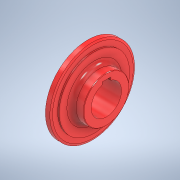
# Autodesk Inventor part: звездочка
Saved by Autodesk Inventor 2021 (Build 250183000, 183)
## iProperties
Created: 2023-04-24
Part Number: звездочка
Material: Сталь, углеродистая
Document SubType Name: Modeling
Designer: gdevc
Density: 7.85 g/cm^3
Appearance: Светло-красный
Mass: 4605.53 g
Surface Area: 813.785 cm^2
Volume: 586.691 cm^3
Author: gdevc
Autodesk Inventor part; units mm, degrees
ref_plane "YZ Plane" through (0, 0, 0) normal (1, 0, 0) x (0, 1, 0)
ref_plane "XY Plane" through (0, 0, 0) normal (0, 0, 1) x (1, 0, 0)
sketch "Эскиз1" plane through (0, 0, 0) normal (0, 0, 1) x (1, 0, 0)
  line L0 (0, 32.5) -> (70, 32.5)
  line L1 (0, 0) -> (109.6934, 0)
  line L2 (0, 32.5) -> (0, 44.804)
  line L3 (35, 68.0113) -> (35, 17.7812) construction
  line L4 (0, 80) -> (70, 80) construction
  line L5 (70, 32.5) -> (0, 32.5)
  line L6 (70, 32.5) -> (70, 44.804)
  line L7 (35, 68.0113) -> (35, 105.8973) construction
  line L8 (35, 90.75) -> (30.3125, 90.75)
  line L9 (30.3125, 90.75) -> (32.3125, 90.75) construction
  line L10 (35, 86.4571) -> (28.75, 86.4571)
  line L11 (30.3125, 90.75) -> (28.75, 86.4571)
  line L12 (28.75, 86.4571) -> (28.75, 75.5)
  line L13 (35, 86.4571) -> (41.25, 86.4571)
  line L14 (39.6875, 90.75) -> (41.25, 86.4571)
  line L15 (41.25, 86.4571) -> (41.25, 75.5)
  line L16 (39.6875, 90.75) -> (35, 90.75)
  line L17 (28.75, 75.5) -> (25.75, 75.5)
  line L18 (25.75, 75.5) -> (25.75, 72.7004)
  line L19 (25.75, 72.7004) -> (25.75, 58.75)
  arc A0 (15.75, 48.75) -> (25.75, 58.75) centre (15.75, 58.75) ccw
  line L20 (35, 90.75) -> (39.6875, 90.75)
  line L21 (35, 86.4571) -> (41.25, 86.4571)
  line L22 (39.6875, 90.75) -> (41.25, 86.4571)
  line L23 (41.25, 86.4571) -> (41.25, 75.5)
  line L24 (44.25, 75.5) -> (44.25, 72.7004)
  line L25 (44.25, 72.7004) -> (44.25, 58.75)
  arc A1 (44.25, 58.75) -> (54.25, 48.75) centre (54.25, 58.75) ccw
  line L26 (44.25, 75.5) -> (41.25, 75.5)
  line L27 (15.75, 48.75) -> (0, 48.75)
  line L28 (0, 48.75) -> (0, 44.804)
  line L29 (54.25, 48.75) -> (70, 48.75)
  line L30 (70, 48.75) -> (70, 43.7446)
  point P0 (0, 46.804)
  point P1 (12.5, 90.75)
  point P2 (57.5, 90.75)
  point P3 (70, 46.804)
  point P4 (57.5, 90.75)
  point P5 (25.75, 42.5)
  dimension "d0" = 65
  dimension "d1" = 70
  dimension "d2" = 160
  dimension "d9" = 45
  dimension "d10" = 70
  dimension "d15" = 2
  dimension "d18" = 2
  dimension "d28" = 4.6875
  dimension "d31" = 6.25
  dimension "d32" = 70
  dimension "d34" = 181.5
  dimension "d35" = 3
  dimension "d36" = 10
  constraints: 62 end point, 11 symmetric about line, 9 point on line, 7 horizontal, 4 point on circle, 4 vertical, 3 perpendicular, 2 centre point, 1 collinear, 1 tangent, 1 other
  measures "d0" diameter of L0 L1
  measures "d1" distance of L0.start L0.end
  measures "d2" diameter of L4 L1
  measures "d9" distance of point (12.5, 90.75) point (57.5, 90.75)
  measures "d10" distance between parallel lines of L2 L6
  measures "d15" distance of L2.end point (0, 46.804)
  measures "d18" distance of L6.end point (70, 46.804)
  measures "d28" distance of L8.start L8.end
  measures "d31" distance of L10.start L10.end
  measures "d32" angle of L10 L11
  measures "d34" diameter of L16 L1
  measures "d35" distance of L12.end L17.end
  measures "d36" radius of A0
ref_plane "РабПлоскость1" through (0, 32.5, 0) normal (0, 1, 0) x (-1, 0, 0)
revolve "Вращение2" add sketch "Эскиз1" angle 360 about axis through (0, 0, 0) along (1, 0, 0)
sketch "Эскиз2" plane through (0, 32.5, 0) normal (0, 1, 0) x (-1, 0, 0)
  line L0 (-70, -8.9471) -> (0, -8.9471)
  line L1 (0, -8.9471) -> (0, 9.0529)
  line L2 (0, 9.0529) -> (-70, 9.0529)
  line L3 (-70, 9.0529) -> (-70, -8.9471)
  line L4 (-70, 32.5) -> (-70, -32.5) projected
  point P0 (0, 0)
  dimension "d21" = 18
  dimension "d22" = 0
  dimension "d23" = 70
  constraints: 8 end point, 2 parallel, 1 horizontal, 1 perpendicular
  measures "d21" distance between parallel lines of L2 L0
  measures "d22" distance between parallel lines of L4 L3
  measures "d23" distance between parallel lines of L1 L3
extrude "Выдавливание1" cut sketch "Эскиз2" along normal blind 4.4 and the other way blind 19.45
chamfer "Фаска1" distance 1 angle 45 2 edges at (0, -48.75, 0) (70, -48.75, 0)
equation "\"d15\" = d11"
equation "\"d18\" = d17"
equation "\"d17\" = d11"
equation "\"d11\" = 2"
